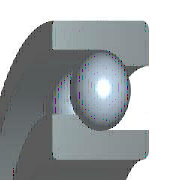
# Autodesk Inventor part: SKF B7202 BE
Saved by Autodesk Inventor 2018 (Build 220112000, 112)
## iProperties
Created: 2017-02-09
Part Number: SKF B7202 BE
Material: Acciaio, Dolce
Description: Cuscinetto a sfere, contatto angolare SKF
Document SubType Name: Modeling
Standard: SKF B
Designer: Francesco
Language: it-IT
Size Designation: SKF B7202 BE
Categories: <MemberInstance><Categories><Category DisplayName="Parti albero" InternalName="7f7aeb1f-a693-4053-b835-cee3144e0d98" Mnemonic="SHFT"><Category DisplayName="Cuscinetti" InternalName="242d30a3-7172-44e6-a363-b0a3d8f1b556" Mnemonic="BRNG"><CategoryParameter DisplayName="Larghezza" InternalName="25fc5f6e-338b-4801-b5ed-8959743e396e" Mnemonic="wdth"/><CategoryParameter DisplayName="Designazione dimensione" InternalName="2c4e891a-c8f4-49ed-a5c1-5131476c6feb" Mnemonic="sizedes"/><CategoryParameter DisplayName="Valore carico dinamico di base" InternalName="440972dd-7009-4861-bd45-69ffbb461423" Mnemonic="bdynlrat"/><CategoryParameter DisplayName="Diametro albero" InternalName="91302473-2833-4451-a660-c5d4a8d6a031" Mnemonic="shaftdia"/><CategoryParameter DisplayName="Angolo di contatto" InternalName="aa21a452-7974-4a55-b5cf-1c2972de2aea" Mnemonic="TouchAngle"/><CategoryParameter DisplayName="Diametro esterno" InternalName="d441686c-04bd-4681-b674-94fbc173ec23" Mnemonic="outdia"/><Category DisplayName="Cuscinetti a sfere" InternalName="9b553946-0899-4a5e-a403-c1d9295e77c1" Mnemonic="BALLBEAR"><CategoryParameter DisplayName="Fattore di carico dinamico radiale se Fa/Fr &lt;= e" InternalName="051e59b3-bd55-4dad-8b07-38b5cb912881" Mnemonic="raddynfc1"/><CategoryParameter DisplayName="Valore carico statico di base" InternalName="0f13fbbf-c511-4d43-b4c7-197b47424baf" Mnemonic="bstatlrat"/><CategoryParameter DisplayName="Esponente per determinazione vita utile" InternalName="3029e2ef-9460-4be8-bdfd-dfe61437473d" Mnemonic="lifeexp"/><CategoryParameter DisplayName="Fattore di attrito" InternalName="3086b0f2-3d69-46ff-8a75-fe12e395bb47" Mnemonic="fricfct"/><CategoryParameter DisplayName="Diametro minimo albero" InternalName="4a5be9bc-ad86-4bf2-8167-102dad5d3e27" Mnemonic="minshaftdia"/><CategoryParameter DisplayName="Fattore di carico dinamico assiale se Fa/Fr &gt; e" InternalName="4b6ff741-5956-4a40-80f5-34eb9259f88c" Mnemonic="axdynfc2"/><CategoryParameter DisplayName="Limitazione lubrificante velocità" InternalName="5237843b-2c8d-46d3-8227-f3e9dd85a12e" Mnemonic="lubgrsp"/><CategoryParameter DisplayName="Limitazione olio velocità" InternalName="60628548-8907-44dc-8e09-603d72f5766f" Mnemonic="oilspd"/><CategoryParameter DisplayName="Fattore carico statico assiale" InternalName="74dbf5e2-8362-409a-802f-3c2235668d99" Mnemonic="axdynfc0"/><CategoryParameter DisplayName="Massa" InternalName="7b80f85c-da81-4dea-b8db-d7c689da91b2" Mnemonic="mass"/><CategoryParameter DisplayName="Raggio" InternalName="83352640-dfae-4cba-bc9f-11ecbfb0001c" Mnemonic="rad"/><CategoryParameter DisplayName="Fattore carico statico radiale" InternalName="83ce084d-c51e-4598-a871-e8e1e34b26ee" Mnemonic="raddynfc0"/><CategoryParameter DisplayName="Fattore di carico dinamico assiale se Fa/Fr &lt;= e" InternalName="ae45a7db-08df-4411-99a8-2f035015bff9" Mnemonic="axdynfc1"/><CategoryParameter DisplayName="Diametro incremento mozzo massimo" InternalName="b5cf89e0-ca87-439c-b08c-a25e2999ab06" Mnemonic="maxhubdia"/><CategoryParameter DisplayName="Limitazione valore per determinazione fattore" InternalName="be0ce6fc-cad4-4218-b484-c34dd2571812" Mnemonic="limvalfac"/><CategoryParameter DisplayName="Fattore di carico dinamico radiale se Fa/Fr &gt; e" InternalName="e513bdb7-139f-4b3c-af32-49e0ba1226b9" Mnemonic="raddynfc2"/><CategoryParameter DisplayName="Raggio raccordo incremento massimo" InternalName="f6ce6695-cf2c-4ec9-8d20-66671e0e35a4" Mnemonic="maxstprad"/><Category DisplayName="Cuscinetti a sfere a contatto angolare" InternalName="0b8e5904-7bca-4d33-b75b-fd5460312790" Mnemonic="BBACBB"/></Category></Category></Category><Category DisplayName="TipoDati" InternalName="23b78d0f-2648-40c6-8793-ca6db495c9e8" Mnemonic="DATATYPE"><CategoryParameter DisplayName="NomeVisualizzazione" InternalName="05415f3d-3907-474b-a020-eb9d644f4cf3" Mnemonic="DISPLAYNAME"/><CategoryParameter DisplayName="Norme" InternalName="0c0a119c-1e12-4c84-803f-101930972f5e" Mnemonic="STANDARD"/><CategoryParameter DisplayName="Descrizione" InternalName="13903e3d-64b1-4950-80da-f627842ea37f" Mnemonic="DESCRIPTION"/><CategoryParameter DisplayName="Designazione" InternalName="2675968c-4ce5-49e0-a4f5-552d29089031" Mnemonic="DESIGNATION"/><CategoryParameter DisplayName="Riga di default" InternalName="2af9ec52-faaa-4026-b378-f9fa4afca842" Mnemonic="DEFAULTROW"/><CategoryParameter DisplayName="Nome cartella" InternalName="3f06958e-8713-4116-9be7-ed6184ecc97b" Mnemonic="FOLDERNAME"/><CategoryParameter DisplayName="Guid revisione" InternalName="45a75005-10b1-4dfc-8d6d-dfe629f0b93c" Mnemonic="REVISIONGUID"/><CategoryParameter DisplayName="NomeFile" InternalName="8b46a4cc-9585-4fed-90c3-899f57e09a73" Mnemonic="FILENAME"/><CategoryParameter DisplayName="SocietàNorme" InternalName="8f5914e1-4693-403f-8ab5-d37768198c9d" Mnemonic="STDSORG"/><CategoryParameter DisplayName="Versione famiglia" InternalName="914462f6-6e19-4b14-ba84-155b9680b1d0" Mnemonic="FAMILYREVISION"/><CategoryParameter DisplayName="Revisione norme" InternalName="91d5a463-65c2-4fde-b823-3b7fea5e8e17" Mnemonic="STANDARDREVISION"/><CategoryParameter DisplayName="Revisione membro" InternalName="a65d44b9-392f-4f4f-857b-e4b3d54996fe" Mnemonic="MEMBERREVISION"/><CategoryParameter DisplayName="FormatoPianoRitaglio" InternalName="bc51e27b-3422-4e78-93ef-cec197ddf230" Mnemonic="CLIPFORMAT"/><CategoryParameter DisplayName="Produttore" InternalName="cd6c7a72-a28a-4e50-99a9-2c7f4e13e5ad" Mnemonic="MANUFACTURER"/><CategoryParameter DisplayName="NomeInterno" InternalName="cf1d0246-76d9-4b4a-8305-fa0409afb5c1" Mnemonic="INTERNALNAME"/><CategoryParameter DisplayName="Èmetrico" InternalName="e2385c5b-1ea4-4823-96a8-8de651266ec3" Mnemonic="ISMETRIC"/><Category DisplayName="Parte" InternalName="c0e0b642-3bcb-4cc8-9e80-f96d35c4afa4" Mnemonic="PART"><CategoryParameter DisplayName="Numero parte" InternalName="016b6077-bfbe-49bd-92c9-d8d59c39c941" Mnemonic="PARTNUMBER"/><CategoryParameter DisplayName="Numero di magazzino" InternalName="4dba7c1c-e26c-444e-836c-b08b433409a8" Mnemonic="STOCKNUMBER"/><CategoryParameter DisplayName="Chiave materiale" InternalName="5c9a8adb-dd2b-4535-b97f-0a94a95fe41f" Mnemonic="MATERIALKEY"/><CategoryParameter DisplayName="Materiale" InternalName="818a152a-d3c3-49ca-80ee-df7d91421b8e" Mnemonic="MATERIAL"/></Category></Category><Category DisplayName="DA mappa precedente" InternalName="924fff40-ddd0-4eff-ad42-30e3774ef79e" Mnemonic="LEGACYMAPDA"><CategoryParameter DisplayName="CookieDA" InternalName="316934ee-8fe1-4c7a-9c36-f2d79e1add1a" Mnemonic="DACOOKIE"/></Category><Category DisplayName="MappaPrecedente" InternalName="cd87c42b-3e48-431e-b5c0-1cbeb14dfe77" Mnemonic="LEGACYMAP"><CategoryParameter DisplayName="ID membro DA univoco" InternalName="0918ad47-427f-4fed-ae26-24c81c58f590" Mnemonic="DACOOKIE"/><CategoryParameter DisplayName="Unisci11 ID" InternalName="0ee8fb18-e2ed-4f39-96f6-1f4b5f50aa71" Mnemonic="MERGE11"/><CategoryParameter DisplayName="ID membro CC univoco" InternalName="5193edd4-b2b0-4ab4-9d54-de900eee34e0" Mnemonic="CCCOOKIE"/><CategoryParameter DisplayName="Dividi ID" InternalName="72b5c83c-be7f-45c4-ae51-9160ea6deb26" Mnemonic="SPLIT"/><CategoryParameter DisplayName="IDMembro" InternalName="8e5e0294-fc51-4c8f-b3d7-003dc5ed94f6" Mnemonic="MEMBERID"/><CategoryParameter DisplayName="NomeCatalogo" InternalName="d99d1e27-aa94-4de2-af4c-c348882a6f4f" Mnemonic="CATALOGNAME"/><CategoryParameter DisplayName="NumeroFamiglia" InternalName="e705e1f4-09cb-413e-91f9-551b4188271e" Mnemonic="FAMILYNUMBER"/></Category></Categories><FamilyTemplate Id="N024645A"><FamilyTemplateParameters><FamilyTemplateParameter ObjectType="kUserParameterObject" ValueType="xs:integer" Id="1" ObjectReferenceKey="Diam"/><FamilyTemplateParameter ObjectType="kUserParameterObject" ValueType="xs:integer" Id="2" ObjectReferenceKey="DD"/><FamilyTemplateParameter ObjectType="kUserParameterObject" ValueType="xs:integer" Id="3" ObjectReferenceKey="B"/><FamilyTemplateParameter ObjectType="kUserParameterObject" ValueType="xs:double" Id="4" ObjectReferenceKey="r"/><FamilyTemplateParameter ObjectType="kUserParameterObject" ValueType="xs:double" Id="5" ObjectReferenceKey="r1"/><FamilyTemplateParameter ObjectType="kPropertyObject" ValueType="xs:string" Id="100" ObjectReferenceKey="{32853F0F-3444-11d1-9E93-0060B03C1CA6}" SubObjectId="52"/><FamilyTemplateParameter ObjectType="kPropertyObject" ValueType="xs:string" Id="105" ObjectReferenceKey="{32853F0F-3444-11d1-9E93-0060B03C1CA6}" SubObjectId="5"/><FamilyTemplateParameter ObjectType="kPartComponentDefinitionObject" ValueType="xs:string" Id="110" SubObjectId="Material"/></FamilyTemplateParameters></FamilyTemplate><CategoryParameterMap><ParamToTemplateMap><ParamToTemplate CategoryParameter="//CategoryParameter[@InternalName='05415f3d-3907-474b-a020-eb9d644f4cf3']" ConstantValue="SKF B- Angular contact"/><ParamToTemplate CategoryParameter="//CategoryParameter[@InternalName='cf1d0246-76d9-4b4a-8305-fa0409afb5c1']" ConstantValue="BF24731F-CEAC-4172-B9FF-D946D27A8F0B"/><ParamToTemplate CategoryParameter="//CategoryParameter[@InternalName='3f06958e-8713-4116-9be7-ed6184ecc97b']" ConstantValue="SKF B - angular contact"/><ParamToTemplate CategoryParameter="//CategoryParameter[@InternalName='914462f6-6e19-4b14-ba84-155b9680b1d0']" ConstantValue="10"/><ParamToTemplate CategoryParameter="//CategoryParameter[@InternalName='bc51e27b-3422-4e78-93ef-cec197ddf230']" ConstantValue="CF_INVENTOR.STDPARTS"/><ParamToTemplate CategoryParameter="//CategoryParameter[@InternalName='e2385c5b-1ea4-4823-96a8-8de651266ec3']" ConstantValue="true"/><ParamToTemplate CategoryParameter="//CategoryParameter[@InternalName='13903e3d-64b1-4950-80da-f627842ea37f']" ConstantValue="Single row angular contact ball bearings SKF"/><ParamToTemplate CategoryParameter="//CategoryParameter[@InternalName='8f5914e1-4693-403f-8ab5-d37768198c9d']" TemplateParameter="101"/><ParamToTemplate CategoryParameter="//CategoryParameter[@InternalName='0c0a119c-1e12-4c84-803f-101930972f5e']" ConstantValue="SKF B"/><ParamToTemplate CategoryParameter="//CategoryParameter[@InternalName='cd6c7a72-a28a-4e50-99a9-2c7f4e13e5ad']" TemplateParameter="104"/><ParamToTemplate CategoryParameter="//CategoryParameter[@InternalName='91d5a463-65c2-4fde-b823-3b7fea5e8e17']" TemplateParameter="103"/><ParamToTemplate CategoryParameter="//CategoryParameter[@InternalName='45a75005-10b1-4dfc-8d6d-dfe629f0b93c']" ConstantValue="a4b1a89d-174f-4ef7-bb69-68bb0fc25248"/><ParamToTemplate CategoryParameter="//CategoryParameter[@InternalName='2af9ec52-faaa-4026-b378-f9fa4afca842']" ConstantValue="10"/><ParamToTemplate CategoryParameter="//CategoryParameter[@InternalName='8b46a4cc-9585-4fed-90c3-899f57e09a73']" ConstantValue="SKF B7202 BE"/><ParamToTemplate CategoryParameter="//CategoryParameter[@InternalName='a65d44b9-392f-4f4f-857b-e4b3d54996fe']" ConstantValue="0f32361b-7e13-4c2b-95a1-4f0d2b22c757"/><ParamToTemplate CategoryParameter="//CategoryParameter[@InternalName='0f13fbbf-c511-4d43-b4c7-197b47424baf']" ConstantValue="4800"/><ParamToTemplate CategoryParameter="//CategoryParameter[@InternalName='5237843b-2c8d-46d3-8227-f3e9dd85a12e']" ConstantValue="17000"/><ParamToTemplate CategoryParameter="//CategoryParameter[@InternalName='3086b0f2-3d69-46ff-8a75-fe12e395bb47']" ConstantValue="0,002"/><ParamToTemplate CategoryParameter="//CategoryParameter[@InternalName='3029e2ef-9460-4be8-bdfd-dfe61437473d']" ConstantValue="3"/><ParamToTemplate CategoryParameter="//CategoryParameter[@InternalName='4a5be9bc-ad86-4bf2-8167-102dad5d3e27']" ConstantValue="20"/><ParamToTemplate CategoryParameter="//CategoryParameter[@InternalName='b5cf89e0-ca87-439c-b08c-a25e2999ab06']" ConstantValue="30"/><ParamToTemplate CategoryParameter="//CategoryParameter[@InternalName='f6ce6695-cf2c-4ec9-8d20-66671e0e35a4']" ConstantValue="0,6"/><ParamToTemplate CategoryParameter="//CategoryParameter[@InternalName='60628548-8907-44dc-8e09-603d72f5766f']" ConstantValue="24000"/><ParamToTemplate CategoryParameter="//CategoryParameter[@InternalName='be0ce6fc-cad4-4218-b484-c34dd2571812']" ConstantValue="1,14"/><ParamToTemplate CategoryParameter="//CategoryParameter[@InternalName='83ce084d-c51e-4598-a871-e8e1e34b26ee']" ConstantValue="0,5"/><ParamToTemplate CategoryParameter="//CategoryParameter[@InternalName='74dbf5e2-8362-409a-802f-3c2235668d99']" ConstantValue="0,26"/><ParamToTemplate CategoryParameter="//CategoryParameter[@InternalName='051e59b3-bd55-4dad-8b07-38b5cb912881']" ConstantValue="1"/><ParamToTemplate CategoryParameter="//CategoryParameter[@InternalName='ae45a7db-08df-4411-99a8-2f035015bff9']" ConstantValue="0"/><ParamToTemplate CategoryParameter="//CategoryParameter[@InternalName='2c4e891a-c8f4-49ed-a5c1-5131476c6feb']" ConstantValue="7202 BE"/><ParamToTemplate CategoryParameter="//CategoryParameter[@InternalName='316934ee-8fe1-4c7a-9c36-f2d79e1add1a']" ConstantValue="*ISO~N024645A~SKF 7202 BE*AFN~N024645A~SKF 7202 BE*ANS~N024645A~SKF 7202 BE*"/><ParamToTemplate CategoryParameter="//CategoryParameter[@InternalName='0918ad47-427f-4fed-ae26-24c81c58f590']" ConstantValue="*ISO~N024645A~SKF 7202 BE*AFN~N024645A~SKF 7202 BE*ANS~N024645A~SKF 7202 BE*"/><ParamToTemplate CategoryParameter="//CategoryParameter[@InternalName='0ee8fb18-e2ed-4f39-96f6-1f4b5f50aa71']" ConstantValue="^644A3735-B5ED-49C0-B3F2-62E0FD95C2D8^EFE989B9-06FC-43C2-B203-6F3548EF0668^B077B6C2-536C-469C-AA3B-E76623965FB8^"/><ParamToTemplate CategoryParameter="//CategoryParameter[@InternalName='25fc5f6e-338b-4801-b5ed-8959743e396e']" TemplateParameter="3"/><ParamToTemplate CategoryParameter="//CategoryParameter[@InternalName='d441686c-04bd-4681-b674-94fbc173ec23']" TemplateParameter="2"/><ParamToTemplate CategoryParameter="//CategoryParameter[@InternalName='2675968c-4ce5-49e0-a4f5-552d29089031']" TemplateParameter="100"/><ParamToTemplate CategoryParameter="//CategoryParameter[@InternalName='91302473-2833-4451-a660-c5d4a8d6a031']" TemplateParameter="1"/><ParamToTemplate CategoryParameter="//CategoryParameter[@InternalName='818a152a-d3c3-49ca-80ee-df7d91421b8e']" TemplateParameter="110"/><ParamToTemplate CategoryParameter="//CategoryParameter[@InternalName='016b6077-bfbe-49bd-92c9-d8d59c39c941']" TemplateParameter="105"/><ParamToTemplate CategoryParameter="//CategoryParameter[@InternalName='83352640-dfae-4cba-bc9f-11ecbfb0001c']" TemplateParameter="4"/></ParamToTemplateMap></CategoryParameterMap></MemberInstance>
Density: 7.85 g/cm^3
Appearance: Semilucidato
IsCustomPart: 0
Author: Francesco
Autodesk Inventor part; units mm, degrees
ref_plane "WorkPlane1" through (0, 0, 0) normal (0, 0, 1) x (1, 0, 0)
ref_plane "Work Plane2" through (0, 0, -11) normal (0, 0, 1) x (1, 0, 0)
ref_plane "WorkPlane2" through (0, 0, 14) normal (0, 0, 1) x (1, 0, 0)
sketch "Schizzo1" plane through (0, 0, 0) normal (-1, 0, 0) x (0, -1, 0)
  point P0 (0, 0)
sketch "Schizzo2" plane through (0, 0, 0) normal (0, 0, 1) x (1, 0, 0)
  point P0 (0, 0)
sketch "Schizzo3" plane through (0, 0, 14) normal (0, 0, 1) x (1, 0, 0)
  point P0 (0, 0)
sketch "Schizzo4" plane through (0, 0, 0) normal (1, 0, 0) x (0, 1, 0)
  line L0 (17.5, 0) -> (7.5, 0)
  line L1 (17.5, 11) -> (17.5, 0)
  line L2 (7.5, 11) -> (17.5, 11)
  line L3 (7.5, 0) -> (7.5, 11)
  line L4 (0, -3.737) -> (0, 15.9311) construction
  line L5 (0, -3.737) -> (0, 15.9311)
  line L6 (0, -7.6706) -> (0, 19.8647) projected
  line L7 (-4.7, 0) -> (28.2, 0) projected
  dimension "d2" = 7.5
  dimension "d4" = 17.5
  dimension "d6" = 11
  constraints: 12 end point, 3 vertical, 2 collinear, 2 horizontal
  measures "d2" horizontal distance of L2.start L4.end
  measures "d4" horizontal distance of L1.start L4.end
  measures "d6" distance of L0.end L2.start
revolve "Rivoluzione1" add sketch "Schizzo4" angle 360 about axis through (0, 0, -3.737) along (0, 0, 1)
sketch "Schizzo5" plane through (0, 0, 0) normal (1, 0, 0) x (0, 1, 0)
  line L0 (15.5, 11) -> (10.7, 11)
  line L1 (15.5, 5.5) -> (15.5, 11)
  arc A0 (14.3, 3.1) -> (15.5, 5.5) centre (12.5, 5.5) ccw
  line L2 (14.3, 0) -> (14.3, 3.1)
  line L3 (9.5, 0) -> (14.3, 0)
  line L4 (9.5, 5.5) -> (9.5, 0)
  arc A1 (10.7, 7.9) -> (9.5, 5.5) centre (12.5, 5.5) ccw
  line L5 (10.7, 11) -> (10.7, 7.9)
  circle A2 centre (12.5, 5.5) radius 3 construction
  line L6 (17.5, 0) -> (-17.5, 0) construction
  line L7 (17.5, 11) -> (-17.5, 11) construction
  line L8 (0, 40.9632) -> (0, -26.9632)
  line L9 (0, -40.5485) -> (0, 54.5485) projected
  dimension "d9" = 5.5
  dimension "d11" = 6
  dimension "d21" = 25
  dimension "d22" = 21.4
  dimension "d23" = 28.6
  constraints: 14 end point, 7 point on circle, 4 vertical, 3 centre point, 3 collinear, 2 horizontal, 2 tangent, 1 coincident, 1 concentric
  measures "d9" vertical distance of A1.centre L2.start
  measures "d11" diameter of A2
  measures "d21" diameter of A0.centre L8
  measures "d22" diameter of L5 L8
  measures "d23" diameter of L2 L8
revolve "Rivoluzione2" cut sketch "Schizzo5" angle 360 about axis through (0, 0, 40.9632) along (0, 0, 1)
sketch "Schizzo6" plane through (0, 0, 0) normal (1, 0, 0) x (0, 1, 0)
  line L0 (12.5, 2.5) -> (12.5, 8.5)
  arc A0 (12.5, 2.5) -> (12.5, 8.5) centre (12.5, 5.5) ccw
  line L1 (12.5, 13.6754) -> (12.5, -2.5126) construction
  line L2 (17.5, 0) -> (-17.5, 0) construction
  line L3 (12.5, 13.6754) -> (12.5, -2.5126)
  arc A1 (10.7, 7.9) -> (9.5, 5.5) centre (12.5, 5.5) ccw projected
  line L4 (15.5, 5.5) -> (-15.5, 5.5) projected
  dimension "d14" = 3
  constraints: 6 end point, 4 point on line, 2 point on circle, 1 centre point, 1 concentric, 1 vertical
  measures "d14" radius of A0
revolve "Rivoluzione3" add sketch "Schizzo6" angle 360 about axis through (0, 12.5, 13.6754) along (0, 0, 1)
pattern_circular "Seriepolare1" count 6 over 360 about axis through (0, 0, 0) along (0, 0, 1) of "Rivoluzione3"
fillet "Raccordo1" radius 0.3 1 edges at (0, -17.5, 11)
fillet "Raccordo2" radius 0.6 3 edges at (0, -17.5, 0) (0, -7.5, 11) (0, -7.5, 0)
equation "\"d19\" = r1"
equation "\"d20\" = r"
equation "\"d2\" = 0.5 * Diam"
equation "\"d4\" = 0.5 * DD"
equation "\"d6\" = B"
equation "\"d9\" = 0.5 * B"
equation "\"d11\" = msp_mdtdk"
equation "\"d21\" = msp_mdtds"
equation "\"d22\" = msp_md"
equation "\"d23\" = msp_vd"
equation "\"d14\" = 0.5 * msp_mdtdk"
equation "\"Diam\" = 15"
equation "\"DD\" = 35"
equation "\"B\" = 11"
equation "\"r\" = 0.6"
equation "\"msp_mdtdk\" = -0.3 * Diam + 0.3 * DD"
equation "\"msp_mdtds\" = 0.5 * DD + 0.5 * Diam"
equation "\"msp_md\" = msp_mdtds - 0.6 * msp_mdtdk"
equation "\"msp_vd\" = msp_mdtds + 0.6 * msp_mdtdk"
equation "\"r1\" = 0.3"
body "Solid1"
